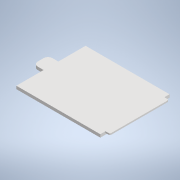
# Autodesk Inventor part: BatteryDoor
Saved by Autodesk Inventor 2022 (Build 260153000, 153)
## iProperties
Created: 2023-09-03
Part Number: BatteryDoor
Material: Generic
Document SubType Name: Modeling
Designer: Petr Černý
Density: 1 g/cm^3
Appearance: Default
Author: Petr Černý
Autodesk Inventor part; units mm, degrees
ref_plane "YZ Plane" through (0, 0, 0) normal (1, 0, 0) x (0, 1, 0)
ref_plane "XZ Plane" through (0, 0, 0) normal (0, 1, 0) x (-1, 0, 0)
ref_plane "XY Plane" through (0, 0, 0) normal (0, 0, 1) x (1, 0, 0)
sketch "Sketch1" plane through (0, 0, 0) normal (0, 1, 0) x (-1, 0, 0)
  line L0 (17.3978, -1.9197) -> (-39.6022, -1.9197)
  line L1 (-39.6022, -1.9197) -> (-39.6022, -48.9197)
  line L2 (-39.6022, -48.9197) -> (17.3978, -48.9197)
  line L3 (17.3978, -48.9197) -> (17.3978, -1.9197)
  point P0 (0, 0)
  dimension "d0" = 47
  dimension "d1" = 57
  constraints: 8 end point, 2 parallel, 1 horizontal, 1 perpendicular
  measures "d0" distance of L2.end L0.start
  measures "d1" distance of L1.end L2.end
extrude "Extrusion1" add sketch "Sketch1" along normal blind 2
sketch "Sketch2" plane through (0, 2, 0) normal (0, 1, 0) x (1, 0, 0)
  line L0 (-17.3978, 48.9197) -> (-17.3978, 1.9197) projected
  line L1 (-17.3978, 20.4197) -> (-21.3978, 20.4197)
  line L2 (-24.3978, 23.4197) -> (-24.3978, 27.4197)
  line L3 (-21.3978, 30.4197) -> (-17.3978, 30.4197)
  line L4 (-17.3978, 30.4197) -> (-17.3978, 20.4197)
  line L5 (-17.3978, 1.9197) -> (39.6022, 1.9197) projected
  arc A0 (-24.3978, 23.4197) -> (-21.3978, 20.4197) centre (-21.3978, 23.4197) ccw
  arc A1 (-21.3978, 30.4197) -> (-24.3978, 27.4197) centre (-21.3978, 27.4197) ccw
  point P0 (0, 0)
  point P1 (-24.3978, 30.4197)
  point P2 (-24.3978, 20.4197)
  dimension "d4" = 10
  dimension "d5" = 18.5
  dimension "d6" = 7
  dimension "d7" = 3
  constraints: 8 end point, 5 point on line, 4 point on circle, 4 tangent, 2 centre point, 2 parallel, 1 equal radius, 1 horizontal, 1 perpendicular
  measures "d4" distance of point (-24.398, 20.42) point (-24.398, 30.42)
  measures "d5" distance between parallel lines of L5 L1
  measures "d6" distance of point (-24.398, 30.42) L3.end
  measures "d7" radius of A0
extrude "Extrusion2" add sketch "Sketch2" against normal blind 2
sketch "Sketch3" plane through (0, 2, 0) normal (0, 1, 0) x (1, 0, 0)
  line L0 (39.6022, 1.9197) -> (39.6022, 48.9197) projected
  line L1 (39.6022, 5.4197) -> (42.6022, 5.4197)
  line L2 (42.6022, 5.4197) -> (42.6022, 45.4197)
  line L3 (42.6022, 45.4197) -> (39.6022, 45.4197)
  line L4 (39.6022, 45.4197) -> (39.6022, 5.4197)
  line L5 (-17.3978, 1.9197) -> (39.6022, 1.9197) projected
  point P0 (0, 0)
  dimension "d10" = 3
  dimension "d11" = 40
  dimension "d12" = 3.5
  constraints: 8 end point, 2 parallel, 1 horizontal, 1 perpendicular, 1 point on line
  measures "d10" distance of L3.end L2.end
  measures "d11" distance of L2.end L1.end
  measures "d12" distance between parallel lines of L5 L1
extrude "Extrusion3" add sketch "Sketch3" against normal blind 1
fillet "Fillet1" radius 1 2 edges at (42.6022, 1.5, -5.4197) (42.6022, 1.5, -45.4197)
body "Solid1"
